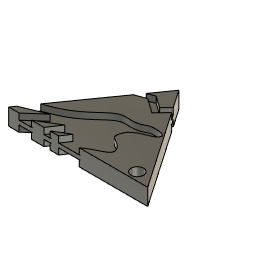
Breloc Corvastch v1 (Autodesk Fusion 360 design; units mm, degrees)
Autodesk Fusion 360 part; units mm, degrees
note: some values were not read from the file. Chosen so that the rebuilt part matches the saved one: which bodies a step acts on.
sketch "Sketch1" plane through (0, 0, 0) normal (0, 0, 1) x (1, 0, 0)
  line L0 (16, -32) -> (49, -32)
  line L1 (49, -32) -> (16, 16)
  line L2 (16, 16) -> (-18, -32)
  line L3 (-18, -32) -> (16, -32)
  line L4 (6.9036, 3.1581) -> (12, 5)
  line L5 (12, 5) -> (18.9151, 0.1018)
  line L6 (18.9151, 0.1018) -> (23.6095, 4.9317)
  line L7 (9.4751, 6.7884) -> (13.0104, 8.0662)
  line L8 (13.0104, 8.0662) -> (18.6393, 4.079)
  line L9 (18.6393, 4.079) -> (21.8937, 7.4273)
  spline S0 degree 5 poles (-11.5783, -22.934) (-11.1719, -22.8047) (-10.3686, -22.5411) (-9.1924, -22.131) (-7.6814, -21.5545) (-5.8884, -20.7848) (-4.1909, -19.9669) (-2.5883, -19.1024) (-1.0791, -18.1949) (0.3395, -17.2494) (1.6718, -16.2734) (2.9238, -15.2771) (4.1036, -14.2738) (5.2212, -13.28) (6.2866, -12.314) (7.3091, -11.3958) (8.2961, -10.5464) (9.2523, -9.7868) (10.1779, -9.138) (11.0689, -8.6194) (11.9234, -8.2438) (12.7462, -8.0133) (13.5537, -7.9151) (14.3813, -7.9154) (15.2737, -7.9654) (16.2655, -8.0123) (17.3668, -8.0088) (18.5423, -7.9244) (19.7096, -7.751) (20.775, -7.4967) (21.6638, -7.1823) (22.3471, -6.8373) (22.8839, -6.495) (23.408, -6.189) (24.0588, -5.9485) (24.9228, -5.7932) (25.9824, -5.7301) (27.1553, -5.7571) (28.3245, -5.867) (29.3686, -6.0505) (30.1971, -6.3) (30.654, -6.5496) (30.8745, -6.7641) (30.9672, -6.9193) (31, -7) knots 0 0 0 0 0 0 0.025 0.05 0.075 0.1 0.125 0.15 0.175 0.2 0.225 0.25 0.275 0.3 0.325 0.35 0.375 0.4 0.425 0.45 0.475 0.5 0.525 0.55 0.575 0.6 0.625 0.65 0.675 0.7 0.725 0.75 0.775 0.8 0.825 0.85 0.875 0.9 0.925 0.95 0.975 1 1 1 1 1 1
  spline S1 degree 5 poles (16, -32) (16.2129, -31.8431) (16.6419, -31.5341) (17.2954, -31.0855) (18.1866, -30.5169) (19.331, -29.8547) (20.4971, -29.2376) (21.6671, -28.6584) (22.8105, -28.1039) (23.8816, -27.5544) (24.814, -26.9803) (25.5327, -26.35) (25.97, -25.6391) (26.079, -24.8387) (25.8511, -23.9663) (25.3259, -23.0702) (24.5738, -22.2108) (23.6834, -21.4452) (22.7478, -20.8116) (21.8505, -20.3104) (21.0551, -19.896) (20.41, -19.4977) (19.9496, -19.0357) (19.6969, -18.4388) (19.6655, -17.6613) (19.8619, -16.6777) (20.2027, -15.7167) (20.5614, -14.8968) (20.8462, -14.3063) (21, -14) knots 0 0 0 0 0 0 0.04 0.08 0.12 0.16 0.2 0.24 0.28 0.32 0.36 0.4 0.44 0.48 0.52 0.56 0.6 0.64 0.68 0.72 0.76 0.8 0.84 0.88 0.92 0.96 1 1 1 1 1 1
  spline S2 degree 5 poles (21, -14) (21.1322, -13.8712) (21.402, -13.6178) (21.8224, -13.2509) (22.4149, -12.7878) (23.2088, -12.2535) (24.054, -11.7636) (24.9442, -11.3167) (25.8673, -10.9084) (26.802, -10.5305) (27.7174, -10.1698) (28.5785, -9.8113) (29.3492, -9.4392) (29.9969, -9.0393) (30.4972, -8.6005) (30.8387, -8.1172) (30.9829, -7.6934) (31.0192, -7.3548) (31.0117, -7.1198) (31, -7) knots 0 0 0 0 0 0 0.066667 0.133333 0.2 0.266667 0.333333 0.4 0.466667 0.533333 0.6 0.666667 0.733333 0.8 0.866667 0.933333 1 1 1 1 1 1
  line L10 (-16.353, -29.6748) -> (-5, -25)
  line L11 (-5, -25) -> (-13, -32)
  line L12 (-7, -32) -> (3, -26)
  line L13 (3, -26) -> (-1, -32)
  line L14 (2, -32) -> (8.8358, -27.8985)
  line L15 (8.8358, -27.8985) -> (6.1015, -32)
  circle A0 centre (40, -28) radius 3
  point P0 (2, -16)
  point P1 (9, -10)
  point P2 (13, -8)
  point P3 (17, -8)
  point P4 (22, -7)
  point P5 (24, -6)
  point P6 (29, -6)
  point P7 (23, -28)
  point P8 (26, -25)
  point P9 (23, -21)
  point P10 (20, -19)
  point P11 (25.5558, -11.0517)
  point P12 (30, -9)
  constraint horizontal L0
  constraint parallel L0 L3
  constraint coincident L2 L4.start
  constraint perpendicular L2 L5
  constraint coincident L1 L6.end
  constraint coincident L2 L7.start
  constraint parallel L4 L7
  constraint perpendicular L2 L8
  constraint coincident L1 L9.end
  constraint parallel L6 L9
  constraint coincident L2 L10.start
  constraint coincident L3 L11.end
  constraint coincident L3 L12.start
  constraint midpoint L3 L13.end
  constraint coincident L3 L14.start
  constraint parallel L12 L14
  constraint coincident L3 L15.end
  constraint parallel L13 L15
extrude "Extrude1" add sketch "Sketch1" along normal mid plane 8 contours L0 L1 L2 L4 L5 L6 S0 S1 S2 | L3 L14 L15 | L1 L2 L7 L8 L9 | L3 L12 L13 | L2 L3 L10 L11 makes body 1 at (-12.5687, -28.1165, 1.3333) makes body 2 at (16.9681, 10.4978, 4) makes body 3 at (-3.6667, -30, 1.3333) makes body 4 at (30.5652, -19.508, 4) makes body 5 at (4.2786, -30.6328, 1.3333)
extrude "Extrude2" add sketch "Sketch1" along normal mid plane 2 contours L2 L3 S0 S1 S2 L10 L11 L12 L13 L14 L15 | L1 L2 L4 L5 L6 L7 L8 L9 bodies 1 2 3 4 5
named bodies: "Breloc"
